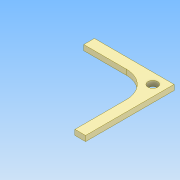
# Autodesk Inventor part: Selection_Selector 1
Saved by Autodesk Inventor 2018.1 (Build 221171000, 171)
## iProperties
Created: 2019-02-14
Part Number: Selection_Selector 1
Material: Nylon 6/6
Document SubType Name: Modeling
Designer: James
Density: 1.13 g/cm^3
Appearance: Nylon 6
Mass: 1.8781 g
Surface Area: 17.1526 cm^2
Volume: 1.66203 cm^3
Author: James
Autodesk Inventor part; units mm, degrees
ref_plane "YZ Plane" through (0, 0, 0) normal (1, 0, 0) x (0, 1, 0)
ref_plane "XZ Plane" through (0, 0, 0) normal (0, 1, 0) x (-1, 0, 0)
ref_plane "XY Plane" through (0, 0, 0) normal (0, 0, 1) x (1, 0, 0)
sketch "Sketch1" plane through (0, 0, 0) normal (0, 0, 1) x (1, 0, 0)
  line L0 (-39, 50) -> (6, 50)
  line L1 (6, 50) -> (6, 44)
  line L2 (6, 44) -> (-39, 44)
  line L3 (-39, 44) -> (-39, 50)
  line L4 (0, 44) -> (6, 44)
  line L5 (6, 44) -> (6, 0)
  line L6 (6, 0) -> (0, 0)
  line L7 (0, 0) -> (0, 44)
  dimension "d1" = 6
  dimension "d2" = 45
  dimension "d3" = 6
  dimension "d17" = 50
  constraints: 16 end point, 4 parallel, 2 coincident, 2 horizontal, 2 perpendicular, 1 point on line
  measures "d1" distance of L0.end L1.end
  measures "d2" distance of L0.start L0.end
  measures "d3" distance of L5.end L6.end
  measures "d17" distance between parallel lines of L6 L0
extrude "Extrusion1" add sketch "Sketch1" along normal blind 3
fillet "Fillet1" radius 15 1 edges at (0, 44, 1.5)
sketch "Sketch2" plane through (0, 0, 3) normal (0, 0, 1) x (1, 0, 0)
  line L0 (6, 50) -> (-39, 50) projected
  line L1 (6, 0) -> (6, 50) projected
  point P0 (0, 0)
  point P1 (0, 44)
  dimension "d8" = 6
  dimension "d9" = 6
  measures "d8" distance from line of point (0, 44) L0
  measures "d9" distance from line of L1 point (0, 44)
hole "Hole1" at (0, 44, 3) direction (0, 0, -1) diameter 5.5 end through all
equation "\"d3\" = d1"
equation "\"d9\" = d8"
body "Solid1"
